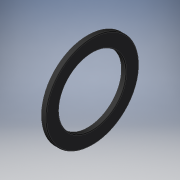
# Autodesk Inventor part: 51110 Shaft washer
Saved by Autodesk Inventor 2019 (Build 230136000, 136)
## iProperties
Created: 2023-07-26
Part Number: 51110 Shaft washer
Material: Generic
Catalog Web Link: www.cadenas.de
Description: With flat seet SW-
Vendor: NSK_RB
Document SubType Name: Modeling
Designer: psAdmin
Manufacturer: NSK_RB
Mass: 7.11095 g
Surface Area: 50.6564 cm^2
Volume: 7.11095 cm^3
Density: 1 g/cm^3
Appearance: PSOLRGB-175-175-175
Category: PARTsolutions
Company: NSK_RB
Title: 51110 Shaft washer
Author: Cadenas PARTsolutions
PSOL_IDENT_0: {$CADENAS_DATA/23d-libs/nsk_rb/roller_bearings/thrust_bearings/single_direction_tbb/with_flat_seet_s
PSOL_IDENT_1: w.prj},189 {VTYP=3D},{NB=51110 Shaft washer},{LINA=51110 Shaft washer},{NN=With flat seet SW},{DATE=
PSOL_IDENT_2: 27.09.2022 23:23:10},{GEOMDATE=23.08.2022 10:45:55},{VERSION=},{LINEID=6550},{WBVAR=},{WBNUMERIC=}
PSOL_IDENT_3: {NB=51110 Shaft washer},{LINA=51110 Shaft washer},{KT=DUMMY},{IDNR=},{STAN=},{NO=31},{ORDER=51110},{
PSOL_IDENT_4: SD=50},{D=70},{T=14},{T3=0.0},{T4=0},{SR=0.6},{CAN=29000},{COAN=75500},{CA=2960},{COA=7700},{GRE=320
PSOL_IDENT_5: 0},{OIL=4800},{SD1=70},{D1=52},{D2=0},{D3=0},{SB=0.0},{A=0.0},{R=0},{SDA=62},{DA=58},{SRA=0.6},{MASS=
PSOL_IDENT_6: 0.153},{N=10},{DIST=2.800}
NB: 51110 Shaft washer
NN: With flat seet SW
NBSYN: $ORDER. Shaft washer
LINA: 51110 Shaft washer
CATALOG: NSK Rolling Bearing
NO: 31
ORDER: 51110
SD: 50
D: 70
T: 14
T3: 0
T4: 0
SR: 0.6
CAN: 29000
COAN: 75500
CA: 2960
COA: 7700
GRE: 3200
OIL: 4800
SD1: 70
D1: 52
D2: 0
D3: 0
SB: 0
A: 0
R: 0
SDA: 62
DA: 58
SRA: 0.6
MASS: 0.153
N: 10
SUPPLIER: NSK_RB
ARTICLENO: 51110 Shaft washer
BOMINFO: 51110 Shaft washer
CREATOR: CADENAS GmbH
Autodesk Inventor part; units mm, degrees
sketch "Sketch_1" plane through (0, 0, 0) normal (0, 0, 1) x (1, 0, 0)
  line L0 (3.8889, 0) -> (0, 0)
  arc A0 (0, 28.8966) -> (0, 32.1034) centre (-3.1111, 30.5) ccw
  line L1 (0, 28.8966) -> (0, 25.6)
  arc A1 (0, 25.6) -> (0.6, 25) centre (0.6, 25.6) ccw
  line L2 (0.6, 25) -> (3.2889, 25)
  arc A2 (3.2889, 25) -> (3.8889, 25.6) centre (3.2889, 25.6) ccw
  line L3 (3.8889, 25.6) -> (3.8889, 34.4)
  arc A3 (3.8889, 34.4) -> (3.2889, 35) centre (3.2889, 34.4) ccw
  line L4 (3.2889, 35) -> (0.6, 35)
  arc A4 (0.6, 35) -> (0, 34.4) centre (0.6, 34.4) ccw
  line L5 (0, 34.4) -> (0, 32.1034)
  constraints: 12 end point, 10 point on circle, 5 centre point
revolve "Revolution1" add sketch "Sketch_1" angle 360 about axis through (3.8889, 0, 0) along (1, 0, 0)
ref_plane "SW_HW_XY" through (-10.1111, 0, 0) normal (1, 0, 0) x (0, 0, -1)
ref_plane "SW_HW_YZ" through (-10.1111, 0, 0) normal (0, 0, -1) x (0, 1, 0)
ref_plane "SW_HW_ZX" through (-10.1111, 0, 0) normal (0, 1, 0) x (1, 0, 0)
body "Solid1"
